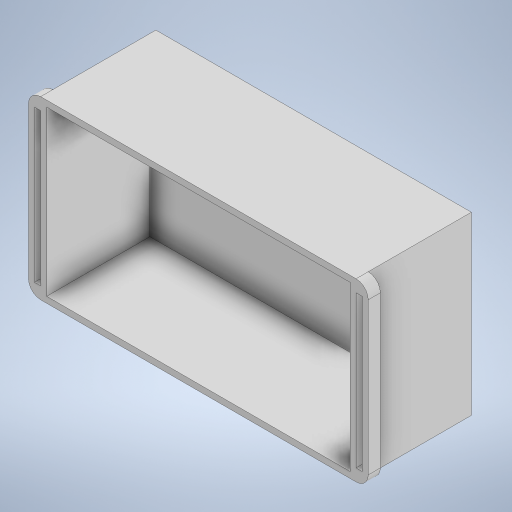
# Autodesk Inventor part: бокс стандартный
Saved by Autodesk Inventor 2023.1 (Build 271208000, 208)
## iProperties
Created: 2023-04-14
Part Number: бокс стандартный
Material: Типовые
Document SubType Name: Modeling
Designer: User
Density: 1 g/cm^3
Appearance: По умолчанию
Author: User
Autodesk Inventor part; units mm, degrees
ref_plane "YZ Plane" through (0, 0, 0) normal (1, 0, 0) x (0, 1, 0)
ref_plane "XZ Plane" through (0, 0, 0) normal (0, 1, 0) x (-1, 0, 0)
ref_plane "XY Plane" through (0, 0, 0) normal (0, 0, 1) x (1, 0, 0)
sketch "Эскиз1" plane through (0, 0, 0) normal (0, 0, 1) x (1, 0, 0)
  line L0 (-26, 14.5) -> (26, 14.5)
  line L1 (26, 14.5) -> (26, -14.5)
  line L2 (26, -14.5) -> (-26, -14.5)
  line L3 (-26, -14.5) -> (-26, 14.5)
  line L4 (0, -20.3) -> (0, 20.3) projected
  line L5 (-36.4, 0) -> (36.4, 0) projected
  point P0 (0, 0)
  dimension "d0" = 29
  dimension "d1" = 52
  constraints: 8 end point, 2 parallel, 1 horizontal, 1 perpendicular, 2 other
  measures "d0" distance between parallel lines of L2 L0
  measures "d1" distance between parallel lines of L1 L3
extrude "Выдавливание1" add sketch "Эскиз1" along normal blind 2
sketch "Эскиз2" plane through (0, 0, 2) normal (0, 0, 1) x (1, 0, 0)
  line L0 (-26, 14.5) -> (-26, -14.5) projected
  line L1 (26, 14.5) -> (-26, 14.5) projected
  line L2 (26, -14.5) -> (26, 14.5) projected
  line L3 (-26, -14.5) -> (26, -14.5) projected
  line L4 (-26, 14.5) -> (26, 14.5)
  line L5 (26, 14.5) -> (26, -14.5)
  line L6 (26, -14.5) -> (-26, -14.5)
  line L7 (-26, -14.5) -> (-26, 14.5)
  line L8 (-25, 13.5) -> (25, 13.5)
  line L9 (25, 13.5) -> (25, -13.5)
  line L10 (25, -13.5) -> (-25, -13.5)
  line L11 (-25, -13.5) -> (-25, 13.5)
  point P0 (0, 0)
  dimension "d4" = 1
  dimension "d5" = 1
  dimension "d6" = 1
  dimension "d7" = 1
  constraints: 16 end point, 4 parallel, 2 horizontal, 2 perpendicular
  measures "d4" distance between parallel lines of L1 L8
  measures "d5" distance between parallel lines of L0 L11
  measures "d6" distance between parallel lines of L3 L10
  measures "d7" distance between parallel lines of L2 L9
extrude "Выдавливание2" add sketch "Эскиз2" along normal blind 15
sketch "Эскиз3" plane through (0, 0, 17) normal (0, 0, 1) x (1, 0, 0)
  line L0 (-26, 14.5) -> (-26, -14.5) projected
  line L1 (-26, 14.5) -> (-26, 14.5)
  line L2 (-26, 14.5) -> (-26, -14.5)
  line L3 (-26, -14.5) -> (-26, -14.5)
  line L4 (-28, -12.5) -> (-28, 12.5)
  line L5 (26, 14.5) -> (-26, 14.5) projected
  line L6 (26, 14.5) -> (26, 14.5)
  line L7 (28, 12.5) -> (28, -12.5)
  line L8 (26, -14.5) -> (26, -14.5)
  line L9 (26, -14.5) -> (26, 14.5)
  arc A0 (-26, 14.5) -> (-28, 12.5) centre (-26, 12.5) ccw
  arc A1 (-28, -12.5) -> (-26, -14.5) centre (-26, -12.5) ccw
  arc A2 (26, -14.5) -> (28, -12.5) centre (26, -12.5) ccw
  arc A3 (28, 12.5) -> (26, 14.5) centre (26, 12.5) ccw
  line L10 (-26, 14.5) -> (26, 14.5)
  line L11 (26, -14.5) -> (26, 14.5) projected
  line L12 (-26, -14.5) -> (26, -14.5)
  line L13 (-26, -12.5) -> (-27, -12.5)
  line L14 (-27, -12.5) -> (-27, 12.5)
  line L15 (-27, 12.5) -> (-26, 12.5)
  line L16 (-26, 12.5) -> (-26, -12.5)
  line L17 (26, 12.5) -> (27, 12.5)
  line L18 (27, 12.5) -> (27, -12.5)
  line L19 (27, -12.5) -> (26, -12.5)
  line L20 (26, -12.5) -> (26, 12.5)
  line L21 (-25, 13.5) -> (25, 13.5) projected
  line L22 (-25, -13.5) -> (-25, 13.5) projected
  line L23 (-25, 13.5) -> (-25, -13.5) projected
  line L24 (-25, -13.5) -> (25, -13.5) projected
  line L25 (25, -13.5) -> (25, 13.5) projected
  line L26 (25, 13.5) -> (-25, 13.5) projected
  point P0 (0, 0)
  point P1 (25, 13.5)
  dimension "d10" = 2
  dimension "d11" = 2
  dimension "d12" = 2
  dimension "d13" = 2
  dimension "d14" = 1
  dimension "d15" = 1
  constraints: 36 end point, 9 tangent, 8 parallel, 8 point on circle, 5 horizontal, 4 centre point, 4 perpendicular, 2 equal radius, 1 point on line
  measures "d10" distance between parallel lines of L7 L9
  measures "d11" distance between parallel lines of L4 L0
  measures "d12" radius of A0
  measures "d13" radius of A1
  measures "d14" distance between parallel lines of L0 L14
  measures "d15" distance between parallel lines of L20 L18
extrude "Выдавливание3" add sketch "Эскиз3" along normal blind 2 contours L5 L9 L12 L0 | L0 L15 L14 L13 A1 L4 A0 | A3 L7 A2 L9 L19 L18 L17
